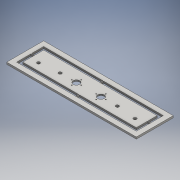
# Autodesk Inventor part: side-UPDATED
Saved by Autodesk Inventor 2016 (Build 200138000, 138)
## iProperties
Created: 2016-10-15
Part Number: side-UPDATED
Material: Generic
Document SubType Name: Modeling
Designer: Kevin G
Density: 1 g/cm^3
Appearance: Default
Author: Kevin G
Autodesk Inventor part; units mm, degrees
ref_plane "YZ Plane" through (0, 0, 0) normal (1, 0, 0) x (0, 1, 0)
ref_plane "XZ Plane" through (0, 0, 0) normal (0, 1, 0) x (-1, 0, 0)
ref_plane "XY Plane" through (0, 0, 0) normal (0, 0, 1) x (1, 0, 0)
sketch "Sketch1" plane through (0, 0, 0) normal (0, 0, 1) x (1, 0, 0)
  line L0 (-270.2344, -114.33) -> (-270.2344, -13.08)
  line L1 (-238, -114.33) -> (-238, -79.405)
  circle A0 centre (-228.9594, -79.405) radius 7.5
  line L2 (-141, -114.33) -> (-141, -69.88)
  circle A1 centre (-133.7094, -69.88) radius 7.5
  circle A2 centre (-54.3344, -69.88) radius 15.875
  circle A3 centre (-54.3344, -46.8612) radius 2.3813
  circle A4 centre (-31.3157, -69.88) radius 2.3813
  circle A5 centre (-77.3532, -69.88) radius 2.3813
  circle A6 centre (-54.3344, -92.8987) radius 2.3813
  line L3 (-270.2344, -13.08) -> (5.175, -13.08)
  line L4 (-270.2344, -114.33) -> (5.1968, -114.33)
  line L5 (280.6281, -114.33) -> (280.6281, -13.08)
  circle A7 centre (239.3531, -79.405) radius 7.5
  circle A8 centre (144.1031, -69.88) radius 7.5
  circle A9 centre (64.7281, -69.88) radius 15.875
  circle A10 centre (64.7281, -46.8612) radius 2.3813
  circle A11 centre (41.7093, -69.88) radius 2.3813
  circle A12 centre (87.7468, -69.88) radius 2.3813
  circle A13 centre (64.7281, -92.8987) radius 2.3813
  line L6 (280.6281, -13.08) -> (5.175, -13.08)
  line L7 (280.6281, -114.33) -> (5.1968, -114.33)
  line L8 (-285.2344, 1.92) -> (295.5844, 1.92)
  line L9 (295.5844, 1.92) -> (295.5844, -129.33)
  line L10 (295.5844, -129.33) -> (-285.2344, -129.33)
  line L11 (-285.2344, -129.33) -> (-285.2344, 1.92)
  line L12 (-59, 1.92) -> (-59, 25.92)
  line L13 (-285.2344, -38) -> (-309.2344, -38)
  line L14 (-43, -129.33) -> (-43, -153.33)
  line L15 (295.5844, -72.2612) -> (319.5844, -72.2612)
  line L16 (-309.2344, 25.92) -> (319.6281, 25.92)
  line L17 (319.6281, 25.92) -> (319.6281, -153.33)
  line L18 (319.6281, -153.33) -> (-309.2344, -153.33)
  line L19 (-309.2344, -153.33) -> (-309.2344, 25.92)
  line L20 (2, -13.08) -> (2, 1.92)
  line L21 (5.175, -13.08) -> (5.175, 1.92)
  line L22 (2, -129.33) -> (2, -114.33)
  line L23 (-285.2344, -56.825) -> (-270.2344, -56.825)
  line L24 (-285.2344, -60) -> (-270.2344, -60)
  line L25 (280.6281, -56.825) -> (295.5844, -56.825)
  line L26 (5.1968, -114.33) -> (5.175, -129.33)
  line L27 (280.6281, -60) -> (295.5844, -60)
  point P0 (0, 0)
  dimension "d3" = 34.925
  dimension "d4" = 15
  dimension "d6" = 44.45
  dimension "d7" = 15
  dimension "d9" = 31.75
  dimension "d11" = 4.7625
  dimension "d13" = 4.7625
  dimension "d15" = 23.0188
  dimension "d16" = 4.7625
  dimension "d18" = 4.7625
  dimension "d23" = 79.375
  dimension "d24" = 41.275
  dimension "d25" = 550.8625
  dimension "d30" = 24
  dimension "d31" = 24
  dimension "d32" = 24
  dimension "d33" = 24
  dimension "d34" = 3.175
  dimension "d36" = 3.175
  dimension "d44" = 15
  dimension "d45" = 15
  constraints: 56 end point, 16 point on line, 14 centre point, 6 perpendicular, 5 horizontal, 5 parallel, 5 vertical, 2 midpoint
  measures "d3" distance of L1.start L1.end
  measures "d4" diameter of A0
  measures "d6" distance of L2.end L2.start
  measures "d7" diameter of A1
  measures "d9" diameter of A2
  measures "d11" diameter of A3
  measures "d13" diameter of A4
  measures "d15" distance of A2.centre A5.centre
  measures "d16" diameter of A5
  measures "d18" diameter of A6
  measures "d23" distance of A8.centre A9.centre
  measures "d24" distance from line of L5 A7.centre
  measures "d25" distance between parallel lines of L0 L5
  measures "d30" distance of L12.end L12.start
  measures "d31" distance of L13.end L13.start
  measures "d32" distance of L14.start L14.end
  measures "d33" distance of L15.start L15.end
  measures "d34" distance between parallel lines of L21 L20
  measures "d36" distance between parallel lines of L24 L23
  measures "d44" diameter of A8
  measures "d45" diameter of A7
extrude "Extrusion1" add sketch "Sketch1" along normal blind 9.525 contours L0 L3 L6 L5 L7 L4 | L24 L11 L23 L0 | L11 L10 L14 L18 L19 L13 | L4 L26 L10 L22 | L20 L8 L21 L3 | L13 L19 L16 L12 L8 L11 | L10 L9 L8 L12 L16 L17 L18 L14 | L5 L25 L9 L27
sketch "Sketch2" plane through (0, 0, 0) normal (0, 0, -1) x (-1, 0, 0)
  circle A0 centre (-64.7281, -69.88) radius 15.875 projected
  circle A1 centre (-64.7281, -69.88) radius 38.1
  circle A2 centre (54.3344, -69.88) radius 15.875 projected
  circle A3 centre (54.3344, -69.88) radius 38.1
  point P0 (0, 0)
  dimension "d40" = 76.2
  dimension "d41" = 76.2
  constraints: 2 centre point, 2 coincident
  measures "d40" diameter of A1
  measures "d41" diameter of A3
emboss "Emboss1" sketch "Sketch2" operation cut depth 3 direction (0, 0, 1)
body "Solid1"
